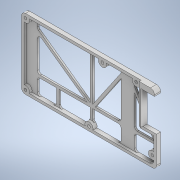
# Autodesk Inventor part: bottom v2 squr
Saved by Autodesk Inventor 2021 (Build 250183000, 183)
## iProperties
Created: 2024-12-22
Part Number: bottom v2 squr
Material: Generic
Document SubType Name: Modeling
Designer: Toby
Density: 1 g/cm^3
Appearance: Default
Author: Toby
Autodesk Inventor part; units mm, degrees
ref_plane "YZ Plane" through (0, 0, 0) normal (1, 0, 0) x (0, 1, 0)
ref_plane "XZ Plane" through (0, 0, 0) normal (0, 1, 0) x (-1, 0, 0)
ref_plane "XY Plane" through (0, 0, 0) normal (0, 0, 1) x (1, 0, 0)
sketch "Sketch1" plane through (0, 0, 0) normal (0, 0, 1) x (1, 0, 0)
  line L0 (-52.3985, 26.3584) -> (47.6015, 26.3584)
  line L1 (47.6015, 26.3584) -> (47.6015, -25.6416)
  line L2 (47.6015, -25.6416) -> (-52.3985, -25.6416)
  line L3 (-52.3985, -25.6416) -> (-52.3985, 26.3584)
  line L4 (-50.3985, 24.3584) -> (45.6015, 24.3584)
  line L5 (45.6015, 24.3584) -> (45.6015, -23.6416)
  line L6 (45.6015, -23.6416) -> (-50.3985, -23.6416)
  line L7 (-50.3985, -23.6416) -> (-50.3985, 24.3584)
  point P0 (0, 0)
  dimension "d0" = 100
  dimension "d1" = 52
  dimension "d2" = 2
  dimension "d3" = 2
  dimension "d4" = 2
  dimension "d5" = 2
  constraints: 16 end point, 4 parallel, 2 horizontal, 2 perpendicular
  measures "d0" distance of L0.start L0.end
  measures "d1" distance of L2.end L0.start
  measures "d2" distance between parallel lines of L4 L0
  measures "d3" distance between parallel lines of L6 L2
  measures "d4" distance between parallel lines of L3 L7
  measures "d5" distance between parallel lines of L1 L5
extrude "Extrusion1" add sketch "Sketch1" along normal blind 3
fillet "Fillet1" radius 3 8 edges at (-50.3985, 24.3584, 1.5) (-52.3985, 26.3584, 1.5) (-50.3985, -23.6416, 1.5) (-52.3985, -25.6416, 1.5) (45.6015, -23.6416, 1.5) (47.6015, -25.6416, 1.5) (45.6015, 24.3584, 1.5) (47.6015, 26.3584, 1.5)
sketch "Sketch2" plane through (0, 0, 0) normal (0, 0, -1) x (-1, 0, 0)
  line L0 (52.3985, 23.3584) -> (52.3985, -22.6416) projected
  line L1 (49.3985, -25.6416) -> (-44.6015, -25.6416) projected
  circle A0 centre (49.3985, 23.3584) radius 3
  circle A1 centre (-7.6015, 23.3584) radius 3
  circle A2 centre (-32.6015, 23.3584) radius 3
  circle A3 centre (2.3985, -22.6416) radius 3
  circle A4 centre (49.3985, -22.6416) radius 3
  circle A5 centre (-44.6015, -17.6416) radius 3
  line L2 (-47.6015, -22.6416) -> (-47.6015, 23.3584) projected
  point P0 (0, 0)
  dimension "d9" = 3
  dimension "d10" = 3
  dimension "d11" = 3
  dimension "d12" = 50
  dimension "d13" = 8
  dimension "d14" = 97
  dimension "d15" = 3
  dimension "d16" = 49
  dimension "d17" = 60
  dimension "d18" = 49
  dimension "d19" = 85
  dimension "d20" = 49
  dimension "d21" = 6
  dimension "d22" = 6
  dimension "d23" = 6
  dimension "d24" = 6
  dimension "d25" = 6
  constraints: 6 centre point, 6 coincident, 1 tangent
  measures "d9" distance from line of L0 point (49.399, -22.642)
  measures "d10" distance from line of L1 point (49.399, -22.642)
  measures "d11" distance from line of L1 point (2.399, -22.642)
  measures "d12" distance from line of L0 point (2.399, -22.642)
  measures "d13" distance from line of L1 point (-44.601, -17.642)
  measures "d14" distance from line of L0 point (-44.601, -17.642)
  measures "d15" distance from line of L0 point (49.399, 23.358)
  measures "d16" distance from line of L1 point (49.399, 23.358)
  measures "d17" distance from line of L0 point (-7.601, 23.358)
  measures "d18" distance from line of L1 point (-7.601, 23.358)
  measures "d19" distance from line of L0 point (-32.601, 23.358)
  measures "d20" distance from line of L1 point (-32.601, 23.358)
  measures "d21" diameter of A0
  measures "d22" diameter of A1
  measures "d23" diameter of A2
  measures "d24" diameter of A3
  measures "d25" diameter of A4
extrude "Extrusion2" add sketch "Sketch2" against normal blind 3
sketch "Sketch3" plane through (0, 0, 0) normal (0, 0, -1) x (-1, 0, 0)
  arc A0 (-35.4299, 24.3584) -> (-29.773, 24.3584) centre (-32.6015, 23.3584) ccw projected
  arc A1 (-10.4299, 24.3584) -> (-4.773, 24.3584) centre (-7.6015, 23.3584) ccw projected
  arc A2 (-45.6015, -20.4701) -> (-45.6015, -14.8132) centre (-44.6015, -17.6416) ccw projected
  arc A3 (5.227, -23.6416) -> (-0.4299, -23.6416) centre (2.3985, -22.6416) ccw projected
  arc A4 (50.3985, -19.8132) -> (46.5701, -23.6416) centre (49.3985, -22.6416) ccw projected
  arc A5 (46.5701, 24.3584) -> (50.3985, 20.5299) centre (49.3985, 23.3584) ccw projected
  point P0 (0, 0)
  constraints: 6 coincident
hole "Hole1" at (32.6015, 23.3584, 0) at (7.6015, 23.3584, 0) at (44.6015, -17.6416, 0) at (-2.3985, -22.6416, 0) at (-49.3985, -22.6416, 0) at (-49.3985, 23.3584, 0) direction (0, 0, 1) diameter 2 depth 4 tip angle 118 countersink diameter 4 countersink angle 90
sketch "Sketch4" plane through (0, 0, 0) normal (0, 0, -1) x (-1, 0, 0)
  line L0 (-42.6015, -23.6416) -> (-0.4299, -23.6416) projected
  arc A0 (5.227, -23.6416) -> (-0.4299, -23.6416) centre (2.3985, -22.6416) ccw projected
  line L1 (46.5701, 24.3584) -> (-4.773, 24.3584) projected
  line L2 (-47.6015, -22.6416) -> (-47.6015, 23.3584) projected
  line L3 (2.3985, -19.6416) -> (2.3985, 24.3584) construction
  line L4 (3.3985, -19.6416) -> (3.3985, 24.3584)
  line L5 (1.3985, 24.3584) -> (1.3985, -19.6416)
  arc A1 (1.3985, -19.6416) -> (3.3985, -19.6416) centre (2.3985, -19.6416) ccw
  arc A2 (3.3985, 24.3584) -> (1.3985, 24.3584) centre (2.3985, 24.3584) ccw
  line L6 (-10.4299, 24.3584) -> (-29.773, 24.3584) projected
  line L7 (-23.6015, 24.3584) -> (-23.6015, -23.6416) construction
  line L8 (-24.6015, 24.3584) -> (-24.6015, -23.6416)
  line L9 (-22.6015, -23.6416) -> (-22.6015, 24.3584)
  arc A3 (-22.6015, 24.3584) -> (-24.6015, 24.3584) centre (-23.6015, 24.3584) ccw
  arc A4 (-24.6015, -23.6416) -> (-22.6015, -23.6416) centre (-23.6015, -23.6416) ccw
  line L10 (-45.6015, 21.3584) -> (-45.6015, -14.8132) projected
  line L11 (49.3985, -25.6416) -> (-44.6015, -25.6416) projected
  line L12 (1.3985, -10.6416) -> (-22.6015, 24.3584) construction
  line L13 (2.2233, -10.0761) -> (-21.7767, 24.9239)
  line L14 (-23.4262, 23.7928) -> (0.5738, -11.2072)
  arc A5 (0.5738, -11.2072) -> (2.2233, -10.0761) centre (1.3985, -10.6416) ccw
  arc A6 (-21.7767, 24.9239) -> (-23.4262, 23.7928) centre (-22.6015, 24.3584) ccw
  line L15 (-24.6015, 24.3584) -> (-45.6015, -10.6416) construction
  line L16 (-25.459, 24.8729) -> (-46.459, -10.1271)
  line L17 (-44.744, -11.1561) -> (-23.744, 23.8439)
  arc A7 (-23.744, 23.8439) -> (-25.459, 24.8729) centre (-24.6015, 24.3584) ccw
  arc A8 (-46.459, -10.1271) -> (-44.744, -11.1561) centre (-45.6015, -10.6416) ccw
  line L18 (50.3985, -19.8132) -> (50.3985, 20.5299) projected
  line L19 (50.3985, -10.6416) -> (2.3985, -10.6416) construction
  line L20 (50.3985, -9.6416) -> (2.3985, -9.6416)
  line L21 (2.3985, -11.6416) -> (50.3985, -11.6416)
  arc A9 (50.3985, -11.6416) -> (50.3985, -9.6416) centre (50.3985, -10.6416) ccw
  arc A10 (2.3985, -9.6416) -> (2.3985, -11.6416) centre (2.3985, -10.6416) ccw
  arc A11 (46.5701, 24.3584) -> (50.3985, 20.5299) centre (49.3985, 23.3584) ccw projected
  line L22 (47.1625, 21.3584) -> (2.3985, -10.6416) construction
  line L23 (46.5809, 22.1719) -> (1.817, -9.8281)
  line L24 (2.9801, -11.4551) -> (47.744, 20.5449)
  arc A12 (47.744, 20.5449) -> (46.5809, 22.1719) centre (47.1625, 21.3584) ccw
  arc A13 (1.817, -9.8281) -> (2.9801, -11.4551) centre (2.3985, -10.6416) ccw
  line L25 (-45.6015, -10.6416) -> (2.3985, -10.6416) construction
  line L26 (-45.6015, -11.6416) -> (2.3985, -11.6416)
  line L27 (2.3985, -9.6416) -> (-45.6015, -9.6416)
  arc A14 (-45.6015, -9.6416) -> (-45.6015, -11.6416) centre (-45.6015, -10.6416) ccw
  arc A15 (2.3985, -11.6416) -> (2.3985, -9.6416) centre (2.3985, -10.6416) ccw
  point P0 (0, 0)
  point P1 (2.3985, 2.3584)
  point P2 (-23.6015, 0.3584)
  point P3 (-10.6015, 6.8584)
  point P4 (-35.1015, 6.8584)
  point P5 (26.3985, -10.6416)
  point P6 (24.7805, 5.3584)
  point P7 (-21.6015, -10.6416)
  point P8 (-22.6015, 22.5901)
  point P9 (-0.4997, -9.6416)
  point P10 (-22.6015, -9.6416)
  point P11 (-24.6015, 22.4147)
  point P12 (-24.6015, -9.6416)
  point P13 (-43.8353, -9.6416)
  point P14 (-25.7677, 24.3584)
  point P15 (-45.6015, -8.698)
  point P16 (-46.459, -10.1271)
  point P17 (-45.6015, -11.6416)
  point P18 (-24.6015, -11.6416)
  point P19 (-22.6015, -11.6416)
  point P20 (1.3985, -11.6416)
  point P21 (1.4125, -19.8083)
  point P22 (3.3845, -19.8083)
  point P23 (3.3985, -11.6416)
  point P24 (5.5169, -9.6416)
  point P25 (3.3985, -8.6975)
  point P26 (1.3985, -8.8734)
  point P27 (-21.389, 24.3584)
  dimension "d35" = 24
  dimension "d36" = 2
  dimension "d37" = 2
  dimension "d38" = 15
  dimension "d39" = 15
  dimension "d40" = 2
  dimension "d41" = 2
  dimension "d42" = 2
  dimension "d43" = 2
  dimension "d44" = 2
  constraints: 56 end point, 32 point on circle, 28 tangent, 14 centre point, 8 point on line, 7 midpoint, 7 parallel, 2 vertical, 1 coincident, 1 concentric, 1 horizontal, 1 perpendicular
  measures "d35" distance from line of L2 L7.end
  measures "d36" diameter of A2
  measures "d37" diameter of A4
  measures "d38" distance from line of L11 L12.start
  measures "d39" distance from line of L11 L15.end
  measures "d40" diameter of A6
  measures "d41" diameter of A8
  measures "d42" diameter of A10
  measures "d43" diameter of A13
  measures "d44" diameter of A15
extrude "Extrusion3" add sketch "Sketch4" against normal blind 1.2 contours L8 L26 L9 L0 | L0 A4 | L26 A8 L17 L27 L8 | L8 L27 L9 L26 | L9 L27 L14 A5 L26 | L8 L17 A7 A6 L14 L9 L27 | A8 A14 L10 | L10 L27 L17 A8 | A1 L5 L26 L21 L4 A0 | A5 L14 L27 L5 | L5 A10 A5 | A5 A10 L26 | L17 L27 L10 L16 L6 L8 | L8 L6 A7 L17 | L14 A6 L6 L9 | L9 L6 L13 L5 L27 L14 | L5 L27 L13 L23 A10 | A10 L13 A5 | A5 L13 A10 A15 A13 | A13 L24 L4 L21 | A3 A7 L6 | L6 A6 A3 | L5 L13 L27 | L23 L13 A10 | L4 L24 L20 L18 L21 | A15 L4 L24 | A7 A3 A6 | L5 L1 L4 L23 L27 L13 | L27 L23 L13 | L13 L23 L27 A10 | L4 L20 L24 | A15 L20 L4 | L23 L4 L20 L27 | L20 L4 L23 A12 A11 L24 | A11 A12
sketch "Sketch5" plane through (0, 0, 0) normal (0, 0, -1) x (-1, 0, 0)
  line L0 (50.3985, -11.6416) -> (3.3985, -11.6416) projected
  line L1 (52.3985, 23.3584) -> (52.3985, -22.6416) projected
  line L2 (5.227, -23.6416) -> (46.5701, -23.6416) projected
  line L3 (27.3985, -11.6416) -> (27.3985, -23.6416) construction
  line L4 (26.3985, -11.6416) -> (26.3985, -23.6416)
  line L5 (28.3985, -23.6416) -> (28.3985, -11.6416)
  arc A0 (28.3985, -11.6416) -> (26.3985, -11.6416) centre (27.3985, -11.6416) ccw
  arc A1 (26.3985, -23.6416) -> (28.3985, -23.6416) centre (27.3985, -23.6416) ccw
  point P0 (0, 0)
  point P1 (27.3985, -17.6416)
  dimension "d47" = 25
  dimension "d48" = 2
  constraints: 8 end point, 4 point on circle, 4 tangent, 2 centre point, 2 point on line, 1 midpoint, 1 parallel, 1 vertical
  measures "d47" distance from line of L1 L3.start
  measures "d48" diameter of A1
extrude "Extrusion4" add sketch "Sketch5" against normal blind 1.2 contours L5 L2 L4 L0
fillet "Fillet2" radius 2 6 edges at (-46.6293, 22.2044, 0.6) (-47.944, 20.7346, 0.6) (-3.3985, 24.3584, 0.6) (-1.3985, 24.3584, 0.6) (21.389, 24.3584, 0.6) (25.7677, 24.3584, 0.6)
fillet "Fillet3" radius 2 6 edges at (-3.3845, -19.8083, 0.6) (-1.4125, -19.8083, 0.6) (-26.3985, -23.6416, 0.6) (-28.3985, -23.6416, 0.6) (24.6015, -23.6416, 0.6) (22.6015, -23.6416, 0.6)
sketch "Sketch6" plane through (0, 0, 3) normal (0, 0, 1) x (1, 0, 0)
  line L0 (44.6015, 26.3584) -> (-49.3985, 26.3584) projected
  line L1 (47.6015, -22.6416) -> (47.6015, 23.3584) projected
  line L2 (35.6015, 26.3584) -> (47.6015, 26.3584)
  line L3 (47.6015, 26.3584) -> (47.6015, -2.6416)
  line L4 (47.6015, -2.6416) -> (35.6015, -2.6416)
  line L5 (35.6015, -2.6416) -> (35.6015, 26.3584)
  point P0 (0, 0)
  dimension "d53" = 12
  dimension "d54" = 29
  constraints: 8 end point, 2 parallel, 2 point on line, 1 horizontal, 1 perpendicular
  measures "d53" distance of L3.end L4.end
  measures "d54" distance from line of L0.start L4
extrude "Extrusion5" cut sketch "Sketch6" against normal blind 10
sketch "Sketch7" plane through (0, 0, 3) normal (0, 0, 1) x (1, 0, 0)
  line L0 (35.6015, 26.3584) -> (35.6015, 24.3584) projected
  line L1 (35.6015, 26.3584) -> (37.6015, 26.3584)
  line L2 (37.6015, 26.3584) -> (37.6015, -2.6416)
  line L3 (37.6015, -2.6416) -> (35.6015, -2.6416)
  line L4 (35.6015, -2.6416) -> (35.6015, 26.3584)
  line L5 (37.6015, -2.6416) -> (47.6015, -2.6416)
  line L6 (47.6015, -2.6416) -> (47.6015, -0.6416)
  line L7 (47.6015, -0.6416) -> (37.6015, -0.6416)
  line L8 (37.6015, -0.6416) -> (37.6015, -2.6416)
  line L9 (47.6015, -22.6416) -> (47.6015, -2.6416) projected
  line L10 (47.6015, -2.6416) -> (45.6015, -2.6416) projected
  point P0 (0, 0)
  dimension "d57" = 2
  dimension "d58" = 2
  constraints: 16 end point, 4 parallel, 2 collinear, 2 horizontal, 2 perpendicular
  measures "d57" distance between parallel lines of L5 L7
  measures "d58" distance between parallel lines of L0 L2
extrude "Extrusion6" add sketch "Sketch7" against normal blind 3
sketch "Sketch8" plane through (0, 0, 3) normal (0, 0, 1) x (1, 0, 0)
  line L0 (37.6015, 26.3584) -> (37.6015, -0.6416) projected
  line L1 (37.6015, 23.3584) -> (36.2015, 23.3584)
  line L2 (36.2015, 23.3584) -> (36.2015, -0.6416)
  line L3 (36.2015, -0.6416) -> (37.6015, -0.6416)
  line L4 (37.6015, -0.6416) -> (37.6015, 23.3584)
  line L5 (36.2015, -0.6416) -> (47.6015, -0.6416)
  line L6 (47.6015, -0.6416) -> (47.6015, -2.0416)
  line L7 (47.6015, -2.0416) -> (36.2015, -2.0416)
  line L8 (36.2015, -2.0416) -> (36.2015, -0.6416)
  line L9 (47.6015, -22.6416) -> (47.6015, -0.6416) projected
  line L10 (47.6015, -0.6416) -> (37.6015, -0.6416) projected
  line L11 (37.6015, 26.3584) -> (-49.3985, 26.3584) projected
  point P0 (0, 0)
  point P1 (34.6015, 26.3584)
  dimension "d62" = 1.4
  dimension "d63" = 1.4
  dimension "d64" = 3
  constraints: 16 end point, 4 collinear, 4 parallel, 2 horizontal, 2 perpendicular, 1 point on line
  measures "d62" distance between parallel lines of L0 L2
  measures "d63" distance between parallel lines of L5 L7
  measures "d64" distance between parallel lines of L1 L11
extrude "Extrusion7" add sketch "Sketch8" along normal blind 1.5
sketch "Sketch9" plane through (0, 0, 0) normal (0, 0, -1) x (-1, 0, 0)
  line L0 (-35.6015, 24.3584) -> (-34.6015, 24.3584)
  line L1 (-34.6015, 24.3584) -> (-34.6015, 20.3584)
  line L2 (-34.6015, 20.3584) -> (-35.6015, 20.3584)
  line L3 (-35.6015, 20.3584) -> (-35.6015, 24.3584)
  line L4 (-34.6015, 20.3584) -> (-32.6015, 20.3584)
  line L5 (-32.6015, 20.3584) -> (-32.6015, 21.3584)
  line L6 (-32.6015, 21.3584) -> (-34.6015, 21.3584)
  line L7 (-34.6015, 21.3584) -> (-34.6015, 20.3584)
  circle A0 centre (-32.6015, 23.3584) radius 1 projected
  line L8 (-35.6015, 7.9687) -> (-35.6015, 23.3584) projected
  line L9 (-35.4299, 24.3584) -> (-35.6015, 24.3584) projected
  point P0 (0, 0)
  dimension "d67" = 3
  dimension "d68" = 1
  dimension "d69" = 1
  dimension "d70" = 3
  constraints: 16 end point, 4 parallel, 2 collinear, 2 horizontal, 2 perpendicular
  measures "d67" distance from line of L4 A0.centre
  measures "d68" distance between parallel lines of L3 L1
  measures "d69" distance between parallel lines of L4 L6
  measures "d70" distance between parallel lines of L3 L5
extrude "Extrusion8" add sketch "Sketch9" against normal blind 2 contours L0 L1 L2 L3 | L6 L5 L4 L1
sketch "Sketch10" plane through (0, 0, 3) normal (0, 0, 1) x (1, 0, 0)
  line L0 (37.6015, 26.3584) -> (-49.3985, 26.3584) projected
  line L1 (36.2015, 23.3584) -> (37.6015, 23.3584) projected
  line L2 (34.6015, 26.3584) -> (37.6015, 26.3584)
  line L3 (37.6015, 26.3584) -> (37.6015, 23.3584)
  line L4 (37.6015, 23.3584) -> (34.6015, 23.3584)
  line L5 (34.6015, 23.3584) -> (34.6015, 26.3584)
  point P0 (0, 0)
  dimension "d73" = 3
  constraints: 8 end point, 2 parallel, 1 horizontal, 1 perpendicular, 1 point on line
  measures "d73" distance between parallel lines of L3 L5
extrude "Extrusion9" add sketch "Sketch10" along normal blind 1.5
fillet "Fillet5" [suppressed]
sketch "Sketch11" plane through (0, 0, 4.5) normal (0, 0, 1) x (1, 0, 0)
  line L0 (34.6015, 26.3584) -> (34.6015, 23.3584) projected
  line L1 (36.2015, 23.3584) -> (35.6015, 23.3584) projected
  line L2 (34.6015, 26.3584) -> (36.2015, 26.3584)
  line L3 (36.2015, 26.3584) -> (36.2015, 23.3584)
  line L4 (36.2015, 23.3584) -> (34.6015, 23.3584)
  line L5 (34.6015, 23.3584) -> (34.6015, 26.3584)
  point P0 (0, 0)
  constraints: 8 end point, 2 parallel, 1 horizontal, 1 perpendicular
extrude "Extrusion10" cut sketch "Sketch11" against normal blind 1.5
sketch "Sketch12" plane through (0, 0, 0) normal (0, 0, -1) x (-1, 0, 0)
  line L0 (-10.4299, 24.3584) -> (-29.773, 24.3584) projected
  line L1 (-42.6015, -23.6416) -> (-0.4299, -23.6416) projected
  line L2 (-29.6015, 24.3584) -> (-19.6015, 24.3584)
  line L3 (-19.6015, 24.3584) -> (-19.6015, -23.6416)
  line L4 (-19.6015, -23.6416) -> (-29.6015, -23.6416)
  line L5 (-29.6015, -23.6416) -> (-29.6015, 24.3584)
  line L6 (-47.6015, -22.6416) -> (-47.6015, -0.6416) projected
  line L7 (-29.6015, 24.3584) -> (-30.6015, 24.3584)
  line L8 (-30.6015, 24.3584) -> (-30.6015, 20.3584)
  line L9 (-30.6015, 20.3584) -> (-29.6015, 20.3584)
  line L10 (-29.6015, 20.3584) -> (-29.6015, 24.3584)
  line L11 (-35.6015, 20.3584) -> (-32.6015, 20.3584) projected
  line L12 (-32.6015, 20.3584) -> (-30.6015, 20.3584)
  line L13 (-30.6015, 20.3584) -> (-30.6015, 21.3584)
  line L14 (-30.6015, 21.3584) -> (-32.6015, 21.3584)
  line L15 (-32.6015, 21.3584) -> (-32.6015, 20.3584)
  point P0 (0, 0)
  dimension "d79" = 10
  dimension "d80" = 18
  dimension "d81" = 1
  dimension "d82" = 1
  dimension "d83" = 3
  constraints: 24 end point, 6 parallel, 4 point on line, 3 horizontal, 3 perpendicular, 1 collinear
  measures "d79" distance between parallel lines of L3 L5
  measures "d80" distance between parallel lines of L6 L5
  measures "d81" distance between parallel lines of L5 L8
  measures "d82" distance between parallel lines of L12 L14
  measures "d83" distance between parallel lines of L10 L15
extrude "Extrusion11" add sketch "Sketch12" against normal blind 1.2
sketch "Sketch13" plane through (0, 0, 0) normal (0, 0, -1) x (-1, 0, 0)
  line L0 (42.3985, 21.3584) -> (50.3985, 21.3584)
  line L1 (50.3985, 21.3584) -> (50.3985, -19.738)
  line L2 (50.3985, -19.738) -> (42.3985, -19.738)
  line L3 (42.3985, -19.738) -> (42.3985, 21.3584)
  line L4 (42.3985, -19.738) -> (47.3985, -19.738)
  line L5 (47.3985, -19.738) -> (47.3985, -23.6416)
  line L6 (47.3985, -23.6416) -> (42.3985, -23.6416)
  line L7 (42.3985, -23.6416) -> (42.3985, -19.738)
  line L8 (52.3985, 23.3584) -> (52.3985, -22.6416) projected
  line L9 (30.3985, -23.6416) -> (46.5701, -23.6416) projected
  line L10 (50.3985, -9.6416) -> (50.3985, 20.5299) projected
  line L11 (-37.6015, 26.3584) -> (49.3985, 26.3584) projected
  line L12 (47.3985, -19.738) -> (50.3985, -19.738)
  line L13 (50.3985, -19.738) -> (50.3985, -20.538)
  line L14 (50.3985, -20.538) -> (47.3985, -20.538)
  line L15 (47.3985, -20.538) -> (47.3985, -19.738)
  line L16 (42.3985, 21.3584) -> (46.8985, 21.3584)
  line L17 (46.8985, 21.3584) -> (46.8985, 24.3584)
  line L18 (46.8985, 24.3584) -> (42.3985, 24.3584)
  line L19 (42.3985, 24.3584) -> (42.3985, 21.3584)
  line L20 (46.5701, 24.3584) -> (5.3985, 24.3584) projected
  point P0 (0, 0)
  point P1 (-34.6015, 26.3584)
  dimension "d86" = 41.0964
  dimension "d87" = 10
  dimension "d88" = 5
  dimension "d89" = 5
  dimension "d90" = 3
  dimension "d91" = 0.8
  dimension "d92" = 4.5
  constraints: 32 end point, 8 parallel, 4 horizontal, 4 perpendicular, 3 collinear
  measures "d86" distance of L2.end L0.start
  measures "d87" distance between parallel lines of L8 L3
  measures "d88" distance between parallel lines of L11 L0
  measures "d89" distance between parallel lines of L8 L5
  measures "d90" distance of L13.end L14.end
  measures "d91" distance of L12.end L13.end
  measures "d92" distance between parallel lines of L19 L17
extrude "Extrusion12" add sketch "Sketch13" against normal blind 1.2
fillet "Fillet6" radius 2 6 edges at (-42.3985, 24.3584, 0.6) (-42.3985, 19.1821, 0.6) (-42.3985, 16.7236, 0.6) (-42.3985, -9.6416, 0.6) (-42.3985, -11.6416, 0.6) (-42.3985, -23.6416, 0.6)
fillet "Fillet7" radius 2 7 edges at (19.6015, -23.6416, 0.6) (29.6015, -23.6416, 0.6) (19.6015, -9.6416, 0.6) (19.6015, -11.6416, 0.6) (29.6015, -11.6416, 0.6) (29.6015, -9.6416, 0.6) (29.6015, 20.3584, 0.6)
sketch "Sketch14" plane through (0, 0, 4.5) normal (0, 0, 1) x (1, 0, 0)
  line L0 (37.6015, -0.6416) -> (47.6015, -0.6416) projected
  line L1 (47.6015, -22.6416) -> (47.6015, -0.6416) projected
  line L2 (37.6015, -0.6416) -> (47.6015, -0.6416)
  line L3 (47.6015, -0.6416) -> (47.6015, -2.6416)
  line L4 (47.6015, -2.6416) -> (37.6015, -2.6416)
  line L5 (37.6015, -2.6416) -> (37.6015, -0.6416)
  line L6 (35.6015, -2.6416) -> (45.6015, -2.6416) projected
  point P0 (0, 0)
  constraints: 8 end point, 2 parallel, 1 collinear, 1 horizontal, 1 perpendicular, 1 point on line
extrude "Extrusion13" cut sketch "Sketch14" against normal blind 5
sketch "Sketch15" plane through (0, 0, 3) normal (0, 0, 1) x (1, 0, 0)
  line L0 (35.6015, -2.6416) -> (37.6015, -2.6416) projected
  line L1 (47.6015, -22.6416) -> (47.6015, -2.6416) projected
  line L2 (35.6015, -2.6416) -> (47.6015, -2.6416)
  line L3 (47.6015, -2.6416) -> (47.6015, -4.6416)
  line L4 (47.6015, -4.6416) -> (35.6015, -4.6416)
  line L5 (35.6015, -4.6416) -> (35.6015, -2.6416)
  point P0 (0, 0)
  dimension "d99" = 2
  constraints: 8 end point, 2 parallel, 1 horizontal, 1 perpendicular, 1 point on line
  measures "d99" distance of L2.end L3.end
extrude "Extrusion14" add sketch "Sketch15" against normal blind 3
sketch "Sketch16" plane through (0, 0, 3) normal (0, 0, 1) x (1, 0, 0)
  line L0 (37.6015, -2.0416) -> (36.2015, -2.0416) projected
  line L1 (37.6015, -2.6416) -> (37.6015, -2.0416) projected
  line L2 (36.2015, -2.0416) -> (37.6015, -2.0416)
  line L3 (37.6015, -2.0416) -> (37.6015, -2.4416)
  line L4 (37.6015, -2.4416) -> (36.2015, -2.4416)
  line L5 (36.2015, -2.4416) -> (36.2015, -2.0416)
  line L6 (47.6015, -2.6416) -> (37.6015, -2.6416) projected
  point P0 (0, 0)
  dimension "d102" = 0.2
  constraints: 8 end point, 2 parallel, 1 horizontal, 1 perpendicular, 1 point on line
  measures "d102" distance between parallel lines of L6 L4
extrude "Extrusion15" add sketch "Sketch16" along normal blind 1.5
sketch "Sketch17" plane through (0, 0, 0) normal (0, 0, -1) x (-1, 0, 0)
  line L0 (-37.6015, -2.4416) -> (-37.6015, 26.3584) projected
  line L1 (-37.6015, 26.3584) -> (-47.6015, 26.3584)
  line L2 (-47.6015, 26.3584) -> (-47.6015, 22.3584)
  line L3 (-47.6015, 22.3584) -> (-37.6015, 22.3584)
  line L4 (-37.6015, 22.3584) -> (-37.6015, 26.3584)
  line L5 (-47.6015, -22.6416) -> (-47.6015, -2.6416) projected
  point P0 (0, 0)
  dimension "d105" = 4
  constraints: 8 end point, 2 parallel, 1 collinear, 1 horizontal, 1 perpendicular
  measures "d105" distance of L1.end L2.end
extrude "Extrusion16" add sketch "Sketch17" against normal blind 4.5
fillet "Fillet8" radius 3 1 edges at (47.6015, 26.3584, 2.25)
body "Solid1"
